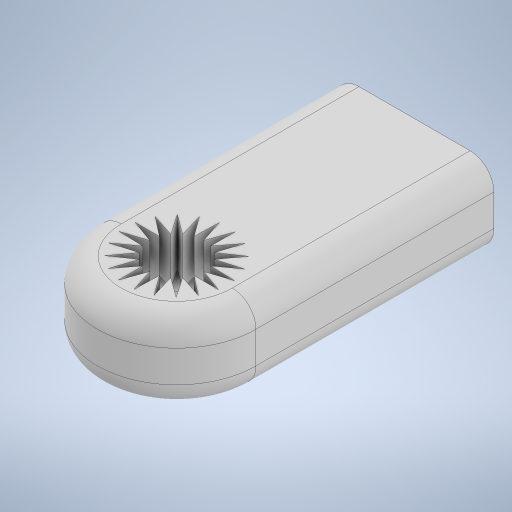
# Autodesk Inventor part: flipper_robot_v2_servo_adapter
Saved by Autodesk Inventor 2023.1 (Build 271208000, 208)
## iProperties
Created: 2025-10-23
Part Number: flipper_robot_v2_servo_adapter
Material: Generic
Document SubType Name: Modeling
Designer: Lars
Density: 1 g/cm^3
Appearance: Default
Author: Lars
Autodesk Inventor part; units mm, degrees
ref_plane "YZ Plane" through (0, 0, 0) normal (1, 0, 0) x (0, 1, 0)
ref_plane "XZ Plane" through (0, 0, 0) normal (0, 1, 0) x (-1, 0, 0)
sketch "Horn Base Profile" plane through (0, 0, 0) normal (0, 1, 0) x (-1, 0, 0)
  line L0 (0, 0) -> (10, 0) construction
  line L1 (10, 0) -> (10, -20) construction
  line L2 (10, -20) -> (0, -20) construction
  line L3 (0, -20) -> (0, 0) construction
  arc A0 (10, -5) -> (0, -5) centre (5, -5) ccw
  line L4 (10, -5) -> (10, -20)
  line L5 (0, -20) -> (10, -20)
  line L6 (0, -20) -> (0, -5)
  circle A1 centre (5, -5) radius 1.5
  dimension "d0" = 10
  dimension "d1" = 20
  dimension "d2" = 3
  constraints: 14 end point, 3 tangent, 2 centre point, 2 collinear, 2 parallel, 2 perpendicular, 2 point on circle, 2 point on line, 1 coincident, 1 horizontal
  measures "d0" distance of L1.end L2.end
  measures "d1" distance of L0.end L1.end
  measures "d2" diameter of A1
extrude "Horn Base" add sketch "Horn Base Profile" along normal blind 2
sketch "Spline Profile" plane through (0, 2, 0) normal (0, 1, 0) x (1, 0, 0)
  line L0 (-10, 20) -> (-10, 5) projected
  arc A0 (-10, 5) -> (0, 5) centre (-5, 5) ccw projected
  line L1 (0, 5) -> (0, 20) projected
  line L2 (0, 20) -> (-10, 20) projected
  circle A1 centre (-5, 5) radius 1.7 construction
  circle A2 centre (-5, 5) radius 3.2 construction
  line L3 (-5, 5) -> (-5, 3.3) construction
  line L4 (-5, 5) -> (-5.5253, 3.3832) construction
  line L5 (-5, 3.3) -> (-5.5253, 1.8434)
  line L6 (-5.5253, 3.3832) -> (-5.5253, 1.8434)
  line L7 (-4.4747, 3.3832) -> (-4.5242, 1.8356)
  line L8 (-5, 3.3) -> (-4.5242, 1.8356)
  line L9 (-4.0008, 3.6247) -> (-3.5696, 2.1375)
  line L10 (-4.4747, 3.3832) -> (-3.5696, 2.1375)
  line L11 (-3.6247, 4.0008) -> (-2.755, 2.7196)
  line L12 (-4.0008, 3.6247) -> (-2.755, 2.7196)
  line L13 (-3.3832, 4.4747) -> (-2.1602, 3.5249)
  line L14 (-3.6247, 4.0008) -> (-2.1602, 3.5249)
  line L15 (-3.3, 5) -> (-1.8434, 4.4747)
  line L16 (-3.3832, 4.4747) -> (-1.8434, 4.4747)
  line L17 (-3.3832, 5.5253) -> (-1.8356, 5.4758)
  line L18 (-3.3, 5) -> (-1.8356, 5.4758)
  line L19 (-3.6247, 5.9992) -> (-2.1375, 6.4304)
  line L20 (-3.3832, 5.5253) -> (-2.1375, 6.4304)
  line L21 (-4.0008, 6.3753) -> (-2.7196, 7.245)
  line L22 (-3.6247, 5.9992) -> (-2.7196, 7.245)
  line L23 (-4.4747, 6.6168) -> (-3.5249, 7.8398)
  line L24 (-4.0008, 6.3753) -> (-3.5249, 7.8398)
  line L25 (-5, 6.7) -> (-4.4747, 8.1566)
  line L26 (-4.4747, 6.6168) -> (-4.4747, 8.1566)
  line L27 (-5.5253, 6.6168) -> (-5.4758, 8.1644)
  line L28 (-5, 6.7) -> (-5.4758, 8.1644)
  line L29 (-5.9992, 6.3753) -> (-6.4304, 7.8625)
  line L30 (-5.5253, 6.6168) -> (-6.4304, 7.8625)
  line L31 (-6.3753, 5.9992) -> (-7.245, 7.2804)
  line L32 (-5.9992, 6.3753) -> (-7.245, 7.2804)
  line L33 (-6.6168, 5.5253) -> (-7.8398, 6.4751)
  line L34 (-6.3753, 5.9992) -> (-7.8398, 6.4751)
  line L35 (-6.7, 5) -> (-8.1566, 5.5253)
  line L36 (-6.6168, 5.5253) -> (-8.1566, 5.5253)
  line L37 (-6.6168, 4.4747) -> (-8.1644, 4.5242)
  line L38 (-6.7, 5) -> (-8.1644, 4.5242)
  line L39 (-6.3753, 4.0008) -> (-7.8625, 3.5696)
  line L40 (-6.6168, 4.4747) -> (-7.8625, 3.5696)
  line L41 (-5.9992, 3.6247) -> (-7.2804, 2.755)
  line L42 (-6.3753, 4.0008) -> (-7.2804, 2.755)
  line L43 (-5.5253, 3.3832) -> (-6.4751, 2.1602)
  line L44 (-5.9992, 3.6247) -> (-6.4751, 2.1602)
  point P0 (0, 0)
  dimension "d5" = 3.4
  dimension "d6" = 1.5
  dimension "d7" = 18
  dimension "d11" = 360
  constraints: 84 end point, 2 point on circle, 2 vertical, 1 centre point, 1 coincident, 104 other
  measures "d5" diameter of A1
  measures "d7" angle of L4 L3
extrude "Servo Spline Cut" add sketch "Spline Profile" along normal blind 3
ref_plane "Work Plane (Clip Axis)" through (0, 2.5, 0) normal (0, 1, 0) x (1, 0, 0)
sketch "Clip Cut Profile" plane through (0, 2.5, 0) normal (0, 1, 0) x (1, 0, 0)
  line L0 (0, 20) -> (-10, 20) construction
  arc A0 (-10, 5) -> (0, 5) centre (-5, 5) ccw construction
  line L1 (0, 5) -> (0, 20) construction
  line L2 (0, 20) -> (-10, 20) construction
  line L3 (-10, 20) -> (-10, 5) construction
  line L4 (-4.4747, 3.3832) -> (-4.5242, 1.8356) construction
  line L5 (-4.5242, 1.8356) -> (-5, 3.3) construction
  line L6 (-5, 3.3) -> (-5.5253, 1.8434) construction
  line L7 (-5.5253, 1.8434) -> (-5.5253, 3.3832) construction
  line L8 (-5.5253, 3.3832) -> (-6.4751, 2.1602) construction
  line L9 (-6.4751, 2.1602) -> (-5.9992, 3.6247) construction
  line L10 (-5.9992, 3.6247) -> (-7.2804, 2.755) construction
  line L11 (-7.2804, 2.755) -> (-6.3753, 4.0008) construction
  line L12 (-6.3753, 4.0008) -> (-7.8625, 3.5696) construction
  line L13 (-7.8625, 3.5696) -> (-6.6168, 4.4747) construction
  line L14 (-6.6168, 4.4747) -> (-8.1644, 4.5242) construction
  line L15 (-8.1644, 4.5242) -> (-6.7, 5) construction
  line L16 (-6.7, 5) -> (-8.1566, 5.5253) construction
  line L17 (-8.1566, 5.5253) -> (-6.6168, 5.5253) construction
  line L18 (-6.6168, 5.5253) -> (-7.8398, 6.4751) construction
  line L19 (-7.8398, 6.4751) -> (-6.3753, 5.9992) construction
  line L20 (-6.3753, 5.9992) -> (-7.245, 7.2804) construction
  line L21 (-7.245, 7.2804) -> (-5.9992, 6.3753) construction
  line L22 (-5.9992, 6.3753) -> (-6.4304, 7.8625) construction
  line L23 (-6.4304, 7.8625) -> (-5.5253, 6.6168) construction
  line L24 (-5.5253, 6.6168) -> (-5.4758, 8.1644) construction
  line L25 (-5.4758, 8.1644) -> (-5, 6.7) construction
  line L26 (-5, 6.7) -> (-4.4747, 8.1566) construction
  line L27 (-4.4747, 8.1566) -> (-4.4747, 6.6168) construction
  line L28 (-4.4747, 6.6168) -> (-3.5249, 7.8398) construction
  line L29 (-3.5249, 7.8398) -> (-4.0008, 6.3753) construction
  line L30 (-4.0008, 6.3753) -> (-2.7196, 7.245) construction
  line L31 (-2.7196, 7.245) -> (-3.6247, 5.9992) construction
  line L32 (-3.6247, 5.9992) -> (-2.1375, 6.4304) construction
  line L33 (-2.1375, 6.4304) -> (-3.3832, 5.5253) construction
  line L34 (-3.3832, 5.5253) -> (-1.8356, 5.4758) construction
  line L35 (-1.8356, 5.4758) -> (-3.3, 5) construction
  line L36 (-3.3, 5) -> (-1.8434, 4.4747) construction
  line L37 (-1.8434, 4.4747) -> (-3.3832, 4.4747) construction
  line L38 (-3.3832, 4.4747) -> (-2.1602, 3.5249) construction
  line L39 (-2.1602, 3.5249) -> (-3.6247, 4.0008) construction
  line L40 (-3.6247, 4.0008) -> (-2.755, 2.7196) construction
  line L41 (-2.755, 2.7196) -> (-4.0008, 3.6247) construction
  line L42 (-4.0008, 3.6247) -> (-3.5696, 2.1375) construction
  line L43 (-3.5696, 2.1375) -> (-4.4747, 3.3832) construction
  line L44 (0, 5) -> (0, 20) construction
  line L45 (0, 20) -> (-10, 20) projected
  line L46 (-5, 20) -> (-6.5, 20)
  line L47 (-6.5, 20) -> (-6.5, 18)
  line L48 (-6.5, 18) -> (-5, 18)
  line L49 (-5, 18) -> (-5, 20)
  line L50 (-5, 18) -> (-7, 18)
  line L51 (-7, 18) -> (-7, 16)
  line L52 (-7, 16) -> (-5, 16)
  line L53 (-5, 16) -> (-5, 18)
  point P0 (0, 0)
  point P1 (-6.5, 18)
  dimension "d16" = 1.5
  dimension "d17" = 2
  dimension "d18" = 2
  dimension "d19" = 2
  constraints: 16 end point, 4 parallel, 2 horizontal, 2 perpendicular, 1 midpoint
  measures "d16" distance of L48.end L47.end
  measures "d17" distance of L47.end L46.end
  measures "d18" distance of L52.end L51.end
  measures "d19" distance of L51.end L50.end
revolve "Fin Clip Cut" cut sketch "Clip Cut Profile" angle 360 about axis through (-5, 2.5, -18) along (0, 0, -1)
fillet "Fillets (Horn Edges)" radius 1.5 6 edges at (-5, 5, 0) (0, 5, -12.5) (-10, 5, -12.5) (-5, 0, 0) (0, 0, -12.5) (-10, 0, -12.5)
body "Solid1"
